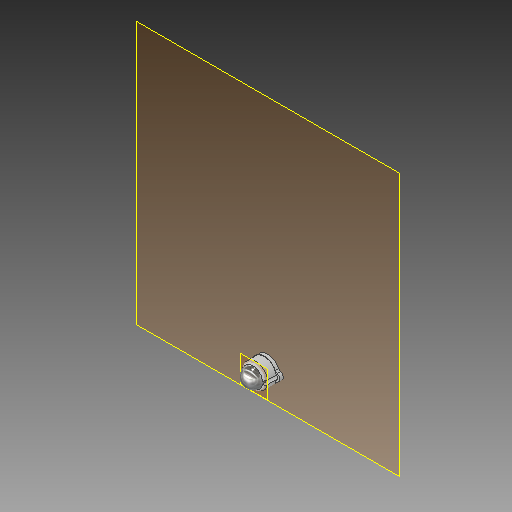
# Autodesk Inventor part: ball
Saved by Autodesk Inventor 2018 (Build 220112000, 112)
## iProperties
Created: 2018-11-21
Part Number: ball
Material: Genérico
Document SubType Name: Modeling
Designer: ivanb
Density: 1 g/cm^3
Appearance: Valor por defecto
Author: ivanb
Autodesk Inventor part; units mm, degrees
ref_plane "YZ Plane" through (0, 0, 0) normal (1, 0, 0) x (0, 1, 0)
ref_plane "XZ Plane" through (0, 0, 0) normal (0, 1, 0) x (-1, 0, 0)
ref_plane "XY Plane" through (0, 0, 0) normal (0, 0, 1) x (1, 0, 0)
ref_plane "Plano de trabajo1" through (0.230933, 0.024747, 0) normal (0, 0, 1) x (1, 0, 0)
sketch "Boceto1" plane through (0.230933, 0.024747, 0) normal (0, 0, 1) x (1, 0, 0)
  circle A0 centre (7.119067, -65.024747) radius 1.25
  circle A1 centre (-7.580933, -65.024747) radius 1.25
  arc A2 (7.015647, -67.522607) -> (7.134973, -62.524797) centre (7.119067, -65.024747) ccw
  arc A3 (-7.596838, -62.524797) -> (-7.477513, -67.522607) centre (-7.580933, -65.024747) ccw
  arc A4 (-7.477513, -67.522607) -> (7.015647, -67.522607) centre (-0.230933, -65.024747) ccw
  arc A5 (7.134973, -62.524797) -> (-7.596838, -62.524797) centre (-0.230933, -65.024747) ccw
  point P0 (-0.230933, -0.024747)
  dimension "d1" = 5
  dimension "d2" = 5
  constraints: 8 point on circle, 4 centre point, 2 coincident
  measures "d1" diameter of A2
  measures "d2" diameter of A3
extrude "Extrusión1" add sketch "Boceto1" along normal blind 2.2
sketch "Boceto2" plane through (0.230933, 0.024747, 2.2) normal (0, 0, 1) x (1, 0, 0)
  circle A0 centre (-7.580933, -65.024747) radius 1.25
  circle A1 centre (7.119067, -65.024747) radius 1.25
  arc A2 (7.015647, -67.522607) -> (7.134973, -62.524797) centre (7.119067, -65.024747) ccw
  arc A3 (7.134973, -62.524797) -> (-7.596838, -62.524797) centre (-0.230933, -65.024747) ccw
  arc A4 (-7.596838, -62.524797) -> (-7.477513, -67.522607) centre (-7.580933, -65.024747) ccw
  arc A5 (-7.477513, -67.522607) -> (7.015647, -67.522607) centre (-0.230933, -65.024747) ccw
  arc A6 (7.334525, -63.793455) -> (-7.79639, -63.793455) centre (-0.230933, -65.024747) ccw
  arc A7 (-7.79639, -66.256038) -> (7.334525, -66.256038) centre (-0.230933, -65.024747) ccw
  point P0 (-0.230933, -0.024747)
  constraints: 8 point on circle, 2 centre point, 1 coincident
extrude "Extrusión2" add sketch "Boceto2" along normal blind 7.21 contours A0 A6 A1 A7 A5
ref_plane "Plano de trabajo2" through (0, -65, 8.852) normal (0, 0, 1) x (-1, 0, 0)
sketch "Boceto3" plane through (0, -65, 8.852) normal (0, 0, 1) x (-1, 0, 0)
  arc A0 (-7.565457, -1.231291) -> (7.565457, -1.231291) centre (0, 0) ccw
  arc A1 (0, 6.35) -> (0, -6.35) centre (0, 0) ccw
  line L0 (0, 6.35) -> (0, -6.35)
  arc A2 (-7.565457, -1.231291) -> (-7.565457, 1.231291) centre (-7.35, 0) ccw
  arc A3 (7.565457, 1.231291) -> (7.565457, -1.231291) centre (7.35, 0) ccw
  arc A4 (7.565457, 1.231291) -> (-7.565457, 1.231291) centre (0, 0) ccw
  point P0 (0, -65)
  dimension "d8" = 12.7
  constraints: 2 end point, 2 point on circle, 1 centre point, 1 coincident, 1 vertical
  measures "d8" diameter of A1
revolve "Revolución1" add sketch "Boceto3" angle 360 about axis through (0, -71.35, 8.852) along (0, 1, 0) contours A2 A1 L0 | A1 A2
fillet "Empalme1" radius 2 1 edges at (0, -57.335, 9.41)
fillet "Empalme2" radius 2 4 edges at (-7.3659, -62.5001, 1.1) (-7.2466, -67.4979, 1.1) (7.2466, -67.4979, 1.1) (7.3659, -62.5001, 1.1)
fillet "Empalme3" radius 2 1 edges at (0, -72.665, 9.41)
